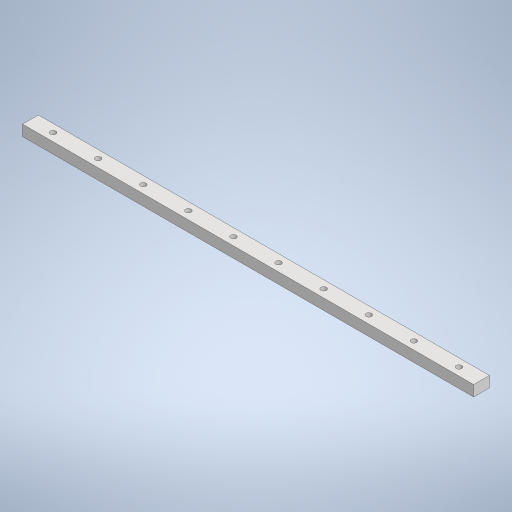
# Autodesk Inventor part: MGN7Cx200mm_rail
Saved by Autodesk Inventor 2024 (Build 280153000, 153)
## iProperties
Created: 2023-08-26
Part Number: MGN7Cx200mm_rail
Material: Generic
Document SubType Name: Modeling
Designer: l1534
Density: 1 g/cm^3
Appearance: Default
Author: l1534
Autodesk Inventor part; units mm, degrees
ref_plane "YZ Plane" through (0, 0, 0) normal (1, 0, 0) x (0, 1, 0)
ref_plane "XZ Plane" through (0, 0, 0) normal (0, 1, 0) x (-1, 0, 0)
ref_plane "XY Plane" through (0, 0, 0) normal (0, 0, 1) x (1, 0, 0)
sketch "Sketch1" plane through (0, 0, 0) normal (1, 0, 0) x (0, 1, 0)
  line L0 (2.1391, 3.4522) -> (-2.6609, 3.4522)
  line L1 (-2.6609, 3.4522) -> (-2.6609, -3.5478)
  line L2 (-2.6609, -3.5478) -> (2.1391, -3.5478)
  line L3 (2.1391, -3.5478) -> (2.1391, 3.4522)
  point P0 (0, 0)
  dimension "d0" = 4.8
  dimension "d1" = 7
  constraints: 8 end point, 2 parallel, 1 horizontal, 1 perpendicular
  measures "d0" distance of L1.end L2.end
  measures "d1" distance of L2.end L0.start
extrude "Extrusion1" add sketch "Sketch1" along normal blind 200
sketch "Sketch2" plane through (0, 2.1391, 3.4522) normal (0, 1, 0) x (1, 0, 0)
  circle A0 centre (10, 3.5) radius 1.2
  line L0 (0, 7) -> (0, 0) projected
  line L1 (0, 0) -> (200, 0) projected
  circle A1 centre (30, 3.5) radius 1.2
  circle A2 centre (50, 3.5) radius 1.2
  circle A3 centre (70, 3.5) radius 1.2
  circle A4 centre (90, 3.5) radius 1.2
  circle A5 centre (110, 3.5) radius 1.2
  circle A6 centre (130, 3.5) radius 1.2
  circle A7 centre (150, 3.5) radius 1.2
  circle A8 centre (170, 3.5) radius 1.2
  circle A9 centre (190, 3.5) radius 1.2
  point P0 (0, 3.4522)
  dimension "d4" = 2.4
  dimension "d5" = 10
  dimension "d6" = 3.5
  dimension "d9" = 20
  constraints: 10 centre point, 1 horizontal, 18 other
  measures "d4" diameter of A0
  measures "d5" distance from line of L0 A0.centre
  measures "d6" distance from line of L1 A0.centre
  measures "d9" distance of A0.centre A1.centre
extrude "Extrusion2" cut sketch "Sketch2" against normal through all
body "Solid1"
